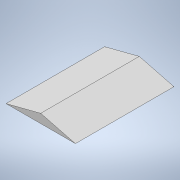
# Autodesk Inventor part: garageRoof
Saved by Autodesk Inventor 2022.1 (Build 261234000, 234)
## iProperties
Created: 2021-07-13
Part Number: garageRoof
Material: Generic
Document SubType Name: Modeling
Designer: robst
Density: 1 g/cm^3
Appearance: Default
Author: robst
Autodesk Inventor part; units mm, degrees
ref_plane "YZ Plane" through (0, 0, 0) normal (1, 0, 0) x (0, 1, 0)
ref_plane "XZ Plane" through (0, 0, 0) normal (0, 1, 0) x (-1, 0, 0)
ref_plane "XY Plane" through (0, 0, 0) normal (0, 0, 1) x (1, 0, 0)
sketch "Sketch1" plane through (0, 0, 0) normal (0, 0, 1) x (1, 0, 0)
  line L0 (0, 0) -> (-6862.8836, 0)
  line L1 (-6862.8836, 0) -> (0, 1766.5584)
  line L2 (0, 1766.5584) -> (0, 0) construction
  line L3 (0, 0) -> (6862.8836, 0)
  line L4 (6862.8836, 0) -> (0, 1766.5584)
  dimension "d0" = 14.435
  dimension "d1" = 14.435
  dimension "d2" = 7086.6
  dimension "d3" = 7086.6
  dimension "d6" = 1766.5584
  constraints: 10 end point, 1 horizontal, 1 perpendicular, 1 point on line
  measures "d0" angle of L1 L0
  measures "d1" angle of L3 L4
  measures "d2" distance of L0.end L1.end
  measures "d3" distance of L3.end L1.end
  measures "d6" distance of L1.end L0.start
extrude "Extrusion1" add sketch "Sketch1" against normal blind 19507.2
equation "\"d0\" = pitch_4_12"
equation "\"d1\" = pitch_4_12"
equation "\"pitch_4_12\" = 14.435deg"
body "Solid1"
